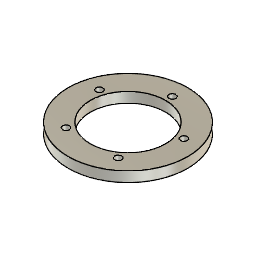
tampa v2 (Autodesk Fusion 360 design; units mm, degrees)
Autodesk Fusion 360 part; units mm, degrees
note: some values were not read from the file. Set by a fixed rule: which sketch regions a step uses.
sketch "Esboço1" plane through (0, 0, 0) normal (0, 0, 1) x (1, 0, 0)
  circle A0 centre (0, 0) radius 175
  line L0 (0, 0) -> (0, 130)
  circle A1 centre (0, 130) radius 10
  circle A2 centre (-123.6373, 40.1722) radius 10
  circle A3 centre (-76.4121, -105.1722) radius 10
  circle A4 centre (76.4121, -105.1722) radius 10
  circle A5 centre (123.6373, 40.1722) radius 10
  dimension "d1" = 350
  dimension "d2" = 130
  dimension "d3" = 20
  dimension "d5" = 360
  constraint coincident A0.centre L0.start
  constraint vertical L0
  constraint coincident L0.end A1.centre
  measures "d1" diameter of A0
  measures "d2" distance of A0.centre L0.end
  measures "d3" diameter of A1
extrude "Extrusão1" add sketch "Esboço1" along normal blind 30
sketch "Sketch2" plane through (0, 0, 30) normal (0, 0, 1) x (-1, 0, 0)
  circle A0 centre (76.4121, 105.1722) radius 10
  circle A1 centre (-123.6373, -40.1722) radius 10
  circle A2 centre (0, -130) radius 10
  circle A3 centre (-76.4121, 105.1722) radius 10
  circle A4 centre (123.6373, -40.1722) radius 10
  circle A5 centre (0, 0) radius 175
  circle A6 centre (0, 0) radius 110
  dimension "d11" = 220
  constraint concentric A5 A6
  measures "d11" diameter of A6
extrude "Extrude2" cut sketch "Sketch2" against normal blind 450 contours A6
